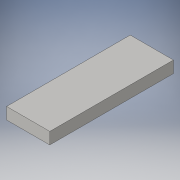
# Autodesk Inventor part: NoiseCan
Saved by Autodesk Inventor 2016 (Build 200138000, 138)
## iProperties
Created: 2016-09-02
Part Number: NoiseCan
Material: Generic
Document SubType Name: Modeling
Designer: jfixelle
Density: 1 g/cm^3
Appearance: Default
Author: jfixelle
Autodesk Inventor part; units mm, degrees
ref_plane "YZ Plane" through (0, 0, 0) normal (1, 0, 0) x (0, 1, 0)
ref_plane "XZ Plane" through (0, 0, 0) normal (0, 1, 0) x (-1, 0, 0)
ref_plane "XY Plane" through (0, 0, 0) normal (0, 0, 1) x (1, 0, 0)
sketch "Sketch1" plane through (0, 0, 0) normal (0, 1, 0) x (-1, 0, 0)
  line L0 (7.366, 21.082) -> (-7.366, 21.082)
  line L1 (-7.366, 21.082) -> (-7.366, -21.082)
  line L2 (-7.366, -21.082) -> (7.366, -21.082)
  line L3 (7.366, -21.082) -> (7.366, 21.082)
  point P0 (0, 0)
  dimension "d0" = 42.164
  dimension "d1" = 21.082
  dimension "d2" = 7.366
  dimension "d3" = 14.732
  constraints: 8 end point, 2 parallel, 1 horizontal, 1 perpendicular
  measures "d0" distance of L2.end L0.start
  measures "d1" distance from line of point (0, 0) L2
  measures "d2" distance from line of point (0, 0) L3
  measures "d3" distance of L0.start L0.end
extrude "Extrusion1" add sketch "Sketch1" along normal blind 4
sketch "Sketch3" plane through (0, 0, 0) normal (0, 1, 0) x (-1, 0, 0)
  line L0 (7.366, 21.082) -> (-7.366, 21.082)
  line L1 (-7.366, 21.082) -> (-7.366, -21.082)
  line L2 (-7.366, -21.082) -> (7.366, -21.082)
  line L3 (7.366, -21.082) -> (7.366, 21.082)
  line L4 (2.534, 19.558) -> (-2.796, 19.558)
  line L5 (-2.796, 19.558) -> (-2.796, 13.714)
  line L6 (-2.796, 13.714) -> (2.534, 13.714)
  line L7 (2.534, 13.714) -> (2.534, 19.558)
  line L8 (5.842, 12.19) -> (-5.842, 12.19)
  line L9 (-5.842, 12.19) -> (-5.842, -3.81)
  line L10 (-5.842, -3.81) -> (5.842, -3.81)
  line L11 (5.842, -3.81) -> (5.842, 12.19)
  line L12 (5.842, -5.334) -> (-5.842, -5.334)
  line L13 (-5.842, -5.334) -> (-5.842, -19.558)
  line L14 (-5.842, -19.558) -> (5.842, -19.558)
  line L15 (5.842, -19.558) -> (5.842, -5.334)
  point P0 (0, 0)
  dimension "d6" = 42.164
  dimension "d7" = 21.082
  dimension "d8" = 14.732
  dimension "d9" = 7.366
  dimension "d10" = 1.524
  dimension "d11" = 1.524
  dimension "d12" = 1.524
  dimension "d13" = 1.524
  dimension "d14" = 1.524
  dimension "d15" = 16
  dimension "d16" = 1.524
  dimension "d17" = 14.224
  dimension "d18" = 1.524
  dimension "d19" = 4.57
  dimension "d20" = 5.33
  constraints: 32 end point, 8 parallel, 4 horizontal, 4 perpendicular, 1 point on line
  measures "d6" distance of L2.end L0.start
  measures "d7" distance from line of L2 point (0, 0)
  measures "d8" distance of L1.end L2.end
  measures "d9" distance from line of point (0, 0) L3
  measures "d10" distance between parallel lines of L3 L11
  measures "d11" distance between parallel lines of L3 L15
  measures "d12" distance between parallel lines of L12 L10
  measures "d13" distance between parallel lines of L2 L14
  measures "d14" distance between parallel lines of L6 L8
  measures "d15" distance of L10.end L8.start
  measures "d16" distance between parallel lines of L0 L4
  measures "d17" distance of L14.end L12.start
  measures "d18" distance between parallel lines of L1 L9
  measures "d19" distance between parallel lines of L1 L5
  measures "d20" distance of L4.start L4.end
extrude "Extrusion2" cut sketch "Sketch3" along normal blind 2 contours L7 L6 L5 L4 | L11 L10 L9 L8 | L15 L14 L13 L12
body "Solid1"
